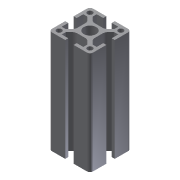
# Autodesk Inventor part: MayTec 1.11.040040.43S_Profile 40x40, 4E, S_100_Detail_(0;0,0,0)
Saved by Autodesk Inventor 2014 (Build 180170000, 170)
## iProperties
Category: PARTsolutions
Company: MAYTEC
Created: 2012-11-14
Part Number: MayTec 1.11.040040.43S_Profile 40x40, 4E, S_100_Detail_(0;0,0,0)
Catalog Web Link: www.cadenas.de
Description: 1.11.040040.43S-Profile 40x40, 4E, S
Vendor: MAYTEC
Document SubType Name: Modeling
Designer: PARTuser1
Manufacturer: MAYTEC
Density: 1 g/cm^3
Material: Generic
Appearance: RGB(175.94999939203154,175.94999939203154,175.94999939203154)
Mass: 134.796 g
Surface Area: 866.32 cm^2
Volume: 134.796 cm^3
PSOL_IDENT_0: {\\10.0.0.242\data_v9\23d-libs\maytec\maytec_3d\profile\profilgruppe_40\40x40\1.11.040040.43s.prj},2
PSOL_IDENT_1: 96 {VTYP=3D},{NB=MayTec 1.11.040040.43S_Profile 40x40, 4E, S_660_Detail_(0;0,0,0)},{LINA=MayTec 1.11
PSOL_IDENT_2: .040040.43S_Profile 40x40, 4E, S_660_Detail_(0;0,0,0)},{NN=1.11.040040.43S},{DATE=14.09.2010 08:41:1
PSOL_IDENT_3: 3},{GEOMDATE=28.01.2010 00:00:00},{VERSION=},{LINEID=10},{LINESUBID=-1},{WBVAR=L,SAX,SAY,EAX,EAY}  {
PSOL_IDENT_4: NB=MayTec 1.11.040040.43S_Profile 40x40, 4E, S_660_Detail_(0;0,0,0)},{LINA=MayTec 1.11.040040.43S_Pr
PSOL_IDENT_5: ofile 40x40, 4E, S_660_Detail_(0;0,0,0)},{KT=DUMMY},{PARTNR=1.11.040040.43S},{DESCRIPTION=Profil 40x
PSOL_IDENT_6: 40, 4E, S},{L=660.0},{DETAIL=Detail},{D=1},{XTRANS=Profile 40x40, 4E, S},{SAX=0},{SAY=0},{EAX=0},{EA
PSOL_IDENT_7: Y=0},{BR=40.0},{HE=40.0},{SDX=0},{EDX=0},{MINLENGTHG=1},{MINLENGTH=50}
CNS_NT: Profile 40x40, 4E, S
CNS_NB: MayTec 1.11.040040.43S_Profile 40x40, 4E, S_660_Detail_(0;0,0,0)
CNS_NBSYN: MayTec $PARTNR._$XTRANS._$L._$DETAIL._($SAX.;$SAY.,$EAX.,$EAY.)
CNS_LINA: MayTec 1.11.040040.43S_Profile 40x40, 4E, S_660_Detail_(0;0,0,0)
CNS_PARTNR: 1.11.040040.43S
CNS_DESCRIPTION: Profile 40x40, 4E, S
CNS_L: 660.0
CNS_DETAIL: Detail
CNS_D: 1
CNS_XTRANS: Profile 40x40, 4E, S
CNS_SAX: 0
CNS_SAY: 0
CNS_EAX: 0
CNS_EAY: 0
CNS_BR: 40.0
CNS_HE: 40.0
CNS_SDX: 0.000
CNS_EDX: 0.000
CNS_MINLENGTHG: 1.000
CNS_MINLENGTH: 50.000
SUPPLIER: MAYTEC
ARTICLENO: MayTec 1.11.040040.43S_Profile 40x40, 4E, S_660_Detail_(0;0,0,0)
BOMINFO: MayTec 1.11.040040.43S_Profile 40x40, 4E, S_660_Detail_(0;0,0,0)
CREATOR: CADENAS GmbH
Title: MayTec 1.11.040040.43S_Profile 40x40, 4E, S_660_Detail_(0;0,0,0)
Author: Cadenas PARTsolutions
Comments: Profile 40x40, 4E, S
Autodesk Inventor part; units mm, degrees
sketch "Skizze_1" plane through (0, 0, 0) normal (0, 0, 1) x (1, 0, 0)
  arc A0 (-20, -17) -> (-17, -20) centre (-17, -17) ccw
  line L0 (-17, -20) -> (-4.1, -20)
  line L1 (-4.1, -20) -> (-4.1, -17)
  line L2 (-4.1, -17) -> (-10.5, -17)
  line L3 (-10.5, -17) -> (-10.5, -13.6627)
  arc A1 (-10.0314, -12.5314) -> (-10.5, -13.6627) centre (-8.9002, -13.6627) ccw
  line L4 (-10.0314, -12.5314) -> (-7.4645, -9.9645)
  arc A2 (-3.9289, -8.5) -> (-7.4645, -9.9645) centre (-3.9289, -13.5) ccw
  line L5 (-3.9289, -8.5) -> (3.9289, -8.5)
  arc A3 (7.4645, -9.9645) -> (3.9289, -8.5) centre (3.9289, -13.5) ccw
  line L6 (7.4645, -9.9645) -> (10.0314, -12.5314)
  arc A4 (10.5, -13.6627) -> (10.0314, -12.5314) centre (8.9002, -13.6627) ccw
  line L7 (10.5, -13.6627) -> (10.5, -17)
  line L8 (10.5, -17) -> (4.1, -17)
  line L9 (4.1, -17) -> (4.1, -20)
  line L10 (4.1, -20) -> (17, -20)
  arc A5 (17, -20) -> (20, -17) centre (17, -17) ccw
  line L11 (20, -17) -> (20, -4.1)
  line L12 (20, -4.1) -> (17, -4.1)
  line L13 (17, -4.1) -> (17, -10.5)
  line L14 (17, -10.5) -> (13.6627, -10.5)
  arc A6 (12.5314, -10.0314) -> (13.6627, -10.5) centre (13.6627, -8.9002) ccw
  line L15 (12.5314, -10.0314) -> (9.9645, -7.4645)
  arc A7 (8.5, -3.9289) -> (9.9645, -7.4645) centre (13.5, -3.9289) ccw
  line L16 (8.5, -3.9289) -> (8.5, 3.9289)
  arc A8 (9.9645, 7.4645) -> (8.5, 3.9289) centre (13.5, 3.9289) ccw
  line L17 (9.9645, 7.4645) -> (12.5314, 10.0314)
  arc A9 (13.6627, 10.5) -> (12.5314, 10.0314) centre (13.6627, 8.9002) ccw
  line L18 (13.6627, 10.5) -> (17, 10.5)
  line L19 (17, 10.5) -> (17, 4.1)
  line L20 (17, 4.1) -> (20, 4.1)
  line L21 (20, 4.1) -> (20, 17)
  arc A10 (20, 17) -> (17, 20) centre (17, 17) ccw
  line L22 (17, 20) -> (4.1, 20)
  line L23 (4.1, 20) -> (4.1, 17)
  line L24 (4.1, 17) -> (10.5, 17)
  line L25 (10.5, 17) -> (10.5, 13.6627)
  arc A11 (10.0314, 12.5314) -> (10.5, 13.6627) centre (8.9002, 13.6627) ccw
  line L26 (10.0314, 12.5314) -> (7.4645, 9.9645)
  arc A12 (3.9289, 8.5) -> (7.4645, 9.9645) centre (3.9289, 13.5) ccw
  line L27 (3.9289, 8.5) -> (-3.9289, 8.5)
  arc A13 (-7.4645, 9.9645) -> (-3.9289, 8.5) centre (-3.9289, 13.5) ccw
  line L28 (-7.4645, 9.9645) -> (-10.0314, 12.5314)
  arc A14 (-10.5, 13.6627) -> (-10.0314, 12.5314) centre (-8.9002, 13.6627) ccw
  line L29 (-10.5, 13.6627) -> (-10.5, 17)
  line L30 (-10.5, 17) -> (-4.1, 17)
  line L31 (-4.1, 17) -> (-4.1, 20)
  line L32 (-4.1, 20) -> (-17, 20)
  arc A15 (-17, 20) -> (-20, 17) centre (-17, 17) ccw
  line L33 (-20, 17) -> (-20, 4.1)
  line L34 (-20, 4.1) -> (-17, 4.1)
  line L35 (-17, 4.1) -> (-17, 10.5)
  line L36 (-17, 10.5) -> (-13.6627, 10.5)
  arc A16 (-12.5314, 10.0314) -> (-13.6627, 10.5) centre (-13.6627, 8.9002) ccw
  line L37 (-12.5314, 10.0314) -> (-9.9645, 7.4645)
  arc A17 (-8.5, 3.9289) -> (-9.9645, 7.4645) centre (-13.5, 3.9289) ccw
  line L38 (-8.5, 3.9289) -> (-8.5, -3.9289)
  arc A18 (-9.9645, -7.4645) -> (-8.5, -3.9289) centre (-13.5, -3.9289) ccw
  line L39 (-9.9645, -7.4645) -> (-12.5314, -10.0314)
  arc A19 (-13.6627, -10.5) -> (-12.5314, -10.0314) centre (-13.6627, -8.9002) ccw
  line L40 (-13.6627, -10.5) -> (-17, -10.5)
  line L41 (-17, -10.5) -> (-17, -4.1)
  line L42 (-17, -4.1) -> (-20, -4.1)
  line L43 (-20, -4.1) -> (-20, -17)
  circle A20 centre (0, 0) radius 6
  constraints: 88 end point, 40 point on circle, 21 centre point
extrude "Extrusion1" add sketch "Skizze_1" against normal blind 100
sketch "Sketch2" plane through (0, 0, 0) normal (0, 0, 1) x (1, 0, 0)
  point P0 (-15, -15)
hole "Drilling 1" at (-15, -15, 0) direction (0, 0, -1) diameter 5 depth 6000
sketch "Sketch3" plane through (0, 0, 0) normal (0, 0, 1) x (1, 0, 0)
  point P0 (15, -15)
hole "Drilling 2" at (15, -15, 0) direction (0, 0, -1) diameter 5 depth 6000
sketch "Sketch4" plane through (0, 0, 0) normal (0, 0, 1) x (1, 0, 0)
  point P0 (15, 15)
hole "Drilling 3" at (15, 15, 0) direction (0, 0, -1) diameter 5 depth 6000
sketch "Sketch5" plane through (0, 0, 0) normal (0, 0, 1) x (1, 0, 0)
  point P0 (-15, 15)
hole "Drilling 4" at (-15, 15, 0) direction (0, 0, -1) diameter 5 depth 6000
ref_plane "side_4d_XY" through (-20, 0, -330) normal (-1, 0, 0) x (0, 1, 0)
ref_plane "side_4d_YZ" through (-20, 0, -330) normal (0, 1, 0) x (0, 0, -1)
ref_plane "side_4d_ZX" through (-20, 0, -330) normal (0, 0, -1) x (-1, 0, 0)
ref_plane "side_1a_XY" through (0, 20, -330) normal (0, 1, 0) x (1, 0, 0)
ref_plane "side_1a_YZ" through (0, 20, -330) normal (1, 0, 0) x (0, 0, -1)
ref_plane "side_1a_ZX" through (0, 20, -330) normal (0, 0, -1) x (0, 1, 0)
ref_plane "side_2b_XY" through (20, 0, -330) normal (1, 0, 0) x (0, -1, 0)
ref_plane "side_2b_YZ" through (20, 0, -330) normal (0, -1, 0) x (0, 0, -1)
ref_plane "side_2b_ZX" through (20, 0, -330) normal (0, 0, -1) x (1, 0, 0)
ref_plane "side_3c_XY" through (0, -20, -330) normal (0, -1, 0) x (-1, 0, 0)
ref_plane "side_3c_YZ" through (0, -20, -330) normal (-1, 0, 0) x (0, 0, -1)
ref_plane "side_3c_ZX" through (0, -20, -330) normal (0, 0, -1) x (0, -1, 0)
ref_plane "end_XY" through (0, 0, -660) normal (0, 0, -1) x (1, 0, 0)
ref_plane "end_YZ" through (0, 0, -660) normal (1, 0, 0) x (0, -1, 0)
ref_plane "end_ZX" through (0, 0, -660) normal (0, -1, 0) x (0, 0, -1)
ref_plane "start_XY" through (0, 0, 0) normal (0, 0, 1) x (1, 0, 0)
ref_plane "start_YZ" through (0, 0, 0) normal (1, 0, 0) x (0, 1, 0)
ref_plane "start_ZX" through (0, 0, 0) normal (0, 1, 0) x (0, 0, 1)
body "Solid1"
